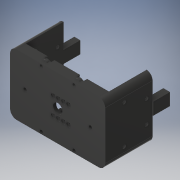
# Autodesk Inventor part: GA03
Saved by Autodesk Inventor 2017 (Build 210142000, 142)
## iProperties
Created: 2018-10-24
Part Number: GA03
Material: ABS Plastic
Document SubType Name: Modeling
Designer: Dell
Density: 1.06 g/cm^3
Appearance: Smooth - Black
Author: Dell
Autodesk Inventor part; units mm, degrees
ref_plane "YZ Plane" through (0, 0, 0) normal (1, 0, 0) x (0, 1, 0)
ref_plane "XZ Plane" through (0, 0, 0) normal (0, 1, 0) x (-1, 0, 0)
ref_plane "XY Plane" through (0, 0, 0) normal (0, 0, 1) x (1, 0, 0)
sketch "Sketch1" plane through (0, 0, 0) normal (0, 0, 1) x (1, 0, 0)
  line L0 (0, 0) -> (150, 0)
  line L1 (150, 0) -> (150, 96.9948)
  line L2 (150, 96.9948) -> (0, 96.9948)
  line L3 (0, 96.9948) -> (0, 0)
  dimension "d0" = 150
  dimension "d1" = 96.9948
  constraints: 8 end point, 2 parallel, 1 horizontal, 1 perpendicular
  measures "d0" distance of L2.end L1.end
  measures "d1" distance of L1.end L0.end
extrude "Extrusion1" add sketch "Sketch1" along normal blind 15
sketch "Sketch2" plane through (0, 0, 0) normal (0, 0, -1) x (-1, 0, 0)
  line L0 (0, 96.9948) -> (0, 0) projected
  line L1 (0, 0) -> (-150, 0) projected
  line L2 (0, 96.9948) -> (-10, 96.9948)
  line L3 (-10, 96.9948) -> (-10, 0)
  line L4 (-10, 0) -> (0, 0)
  line L5 (0, 0) -> (0, 96.9948)
  line L6 (-150, 96.9948) -> (0, 96.9948) projected
  line L7 (-150, 96.9948) -> (-140, 96.9948)
  line L8 (-140, 96.9948) -> (-140, 0)
  line L9 (-140, 0) -> (-150, 0)
  line L10 (-150, 0) -> (-150, 96.9948)
  dimension "d4" = 10
  dimension "d5" = 10
  constraints: 16 end point, 4 parallel, 2 horizontal, 2 perpendicular, 2 point on line
  measures "d4" distance between parallel lines of L3 L0
  measures "d5" distance between parallel lines of L10 L8
extrude "Extrusion2" add sketch "Sketch2" along normal blind 60 contours L0 L1 L3 L2 | L8 L1 L10 L6
sketch "Sketch3" plane through (150, 0, 15) normal (1, 0, 0) x (0, 0, -1)
  circle A0 centre (65, 65.9974) radius 2.5
  circle A1 centre (65, 30.9974) radius 2.5
  line L0 (75, 0) -> (75, 96.9948) projected
  line L1 (65, 65.9974) -> (65, 30.9974) construction
  point P0 (15, 0)
  point P1 (65, 48.4974)
  point P2 (75, 48.4974)
  dimension "d8" = 5
  dimension "d9" = 5
  dimension "d10" = 10
  dimension "d11" = 35
  constraints: 2 centre point, 2 end point, 2 midpoint, 1 horizontal alignment, 1 vertical
  measures "d8" diameter of A0
  measures "d9" diameter of A1
  measures "d10" distance from line of L0 L1.start
  measures "d11" distance of L1.end L1.start
extrude "Extrusion3" cut sketch "Sketch3" against normal through all
sketch "Sketch4" plane through (0, 0, 15) normal (0, 0, 1) x (1, 0, 0)
  line L0 (0, 0) -> (150, 0) projected
  line L1 (150, 0) -> (150, 96.9948) projected
  line L2 (150, 96.9948) -> (0, 96.9948) projected
  line L3 (0, 96.9948) -> (0, 0) projected
  line L4 (149, 1) -> (1, 1)
  line L5 (1, 1) -> (1, 95.9948)
  line L6 (1, 95.9948) -> (149, 95.9948)
  line L7 (149, 95.9948) -> (149, 1)
  dimension "d14" = 1
  constraints: 8 end point, 3 other
  measures "d14" distance between parallel lines of L0 L4
extrude "Extrusion4" cut sketch "Sketch4" against normal through all
sketch "Sketch5" plane through (1, 1, 15) normal (-1, 0, 0) x (0, 0, 1)
  line L0 (-75, 0) -> (-75, 94.9948) projected
  line L1 (-75, 94.9948) -> (-15, 94.9948) projected
  line L2 (-75, 0) -> (-74, 0)
  line L3 (-74, 0) -> (-74, 94.9948)
  line L4 (-74, 94.9948) -> (-75, 94.9948)
  line L5 (-75, 94.9948) -> (-75, 0)
  point P0 (-15, -1)
  dimension "d17" = 1
  constraints: 8 end point, 2 parallel, 1 horizontal, 1 perpendicular, 1 point on line
  measures "d17" distance between parallel lines of L0 L3
extrude "Extrusion5" cut sketch "Sketch5" against normal through all
sketch "Sketch6" plane through (0, 0, 0) normal (0, 0, -1) x (-1, 0, 0)
  line L0 (-10, 95.9948) -> (-140, 95.9948) projected
  line L1 (-140, 95.9948) -> (-140, 1) projected
  line L2 (-140, 1) -> (-10, 1) projected
  line L3 (-10, 1) -> (-10, 95.9948) projected
  line L4 (-15, 6) -> (-135, 6)
  line L5 (-135, 6) -> (-135, 90.9948)
  line L6 (-135, 90.9948) -> (-15, 90.9948)
  line L7 (-15, 90.9948) -> (-15, 6)
  line L8 (-10, 1) -> (-10, 95.9948) projected
  circle A0 centre (-75, 48.4974) radius 2.5
  circle A1 centre (-126, 48.4974) radius 2.5
  circle A2 centre (-100.5, 4.3301) radius 2.5
  circle A3 centre (-49.5, 4.3301) radius 2.5
  circle A4 centre (-24, 48.4974) radius 2.5
  circle A5 centre (-49.5, 92.6647) radius 2.5
  circle A6 centre (-100.5, 92.6647) radius 2.5
  circle A7 centre (-126, 48.4974) radius 5
  circle A8 centre (-100.5, 4.3301) radius 5
  circle A9 centre (-49.5, 4.3301) radius 5
  circle A10 centre (-24, 48.4974) radius 5
  circle A11 centre (-49.5, 92.6647) radius 5
  circle A12 centre (-100.5, 92.6647) radius 5
  point P0 (0, 0)
  point P1 (-75, 6)
  point P2 (-75, 1)
  point P3 (-15, 48.4974)
  point P4 (-10, 48.4974)
  dimension "d20" = 5
  dimension "d21" = 5
  dimension "d22" = 5
  dimension "d23" = 5
  dimension "d26" = 51
  dimension "d29" = 360
  dimension "d31" = 10
  dimension "d34" = 360
  constraints: 13 centre point, 8 end point, 4 midpoint, 3 horizontal alignment, 2 coincident, 2 parallel, 2 vertical alignment, 1 horizontal, 1 perpendicular, 26 other
  measures "d20" distance between parallel lines of L2 L4
  measures "d21" distance between parallel lines of L3 L7
  measures "d22" diameter of A0
  measures "d23" diameter of A1
  measures "d26" distance of A1.centre A0.centre
  measures "d31" diameter of A7
extrude "Extrusion6" cut sketch "Sketch6" against normal blind 10 contours A11 L6 L7 L4 A9 A8 L5 A12 | L6 A5 A11 | A12 L6 A6 | L6 A5 | A9 L4 A3 | A6 L6 | A3 L4 | L4 A2 A8 | L4 A2 | A0 picked at (-49.9702, 90.8634) picked at (-100.0298, 90.8634) picked at (-49.0298, 6.1314) picked at (-100.7933, 6.2234)
extrude "Extrusion7" cut sketch "Sketch6" against normal through all contours A5 L6 | L6 A5 | A6 L6 | L6 A6 | A3 L4 | L4 A3 | A2 L4 | L4 A2 | A1 | A4
extrude "Extrusion8" add sketch "Sketch6" against normal blind 10 contours A11 L6 A5 L0 | L0 A11 | A9 L2 | L2 A9 L4 A3 | A12 L6 A6 L0 | L0 A12 | L6 A5 A11 | A12 L6 A6 | A8 L2 | L2 A8 L4 A2 | A9 L4 A3 | L4 A2 A8
sketch "Sketch7" plane through (0, 0, 10) normal (0, 0, -1) x (-1, 0, 0)
  line L0 (-92, 61.9974) -> (-68, 61.9974) construction
  line L1 (-68, 61.9974) -> (-68, 34.9974) construction
  line L2 (-68, 34.9974) -> (-92, 34.9974) construction
  line L3 (-92, 34.9974) -> (-92, 61.9974) construction
  circle A0 centre (-92, 61.9974) radius 1.5
  circle A1 centre (-92, 34.9974) radius 1.5
  circle A2 centre (-68, 34.9974) radius 1.5
  circle A3 centre (-68, 61.9974) radius 1.5
  circle A4 centre (-84, 61.9974) radius 1.5
  circle A5 centre (-76, 61.9974) radius 1.5
  circle A6 centre (-84, 34.9974) radius 1.5
  circle A7 centre (-76, 34.9974) radius 1.5
  circle A8 centre (-24, 48.4974) radius 2.5 projected
  line L4 (-149, 1) -> (-149, 95.9948) projected
  point P0 (0, 0)
  point P1 (-92, 48.4974)
  point P2 (-80, 61.9974)
  dimension "d42" = 24
  dimension "d43" = 27
  dimension "d44" = 3
  dimension "d45" = 3
  dimension "d46" = 3
  dimension "d47" = 3
  dimension "d48" = 3
  dimension "d49" = 3
  dimension "d50" = 3
  dimension "d51" = 3
  dimension "d52" = 8
  dimension "d53" = 8
  dimension "d55" = 57
  constraints: 8 centre point, 8 end point, 4 coincident, 4 point on line, 2 midpoint, 2 parallel, 2 vertical alignment, 1 horizontal, 1 horizontal alignment, 1 perpendicular
  measures "d42" distance of L2.start L2.end
  measures "d43" distance of L0.end L2.start
  measures "d44" diameter of A0
  measures "d45" diameter of A1
  measures "d46" diameter of A2
  measures "d47" diameter of A3
  measures "d48" diameter of A4
  measures "d49" diameter of A5
  measures "d50" diameter of A6
  measures "d51" diameter of A7
  measures "d52" distance of L2.start A7.centre
  measures "d53" distance of L2.end A6.centre
  measures "d55" distance between parallel lines of L4 L3
extrude "Extrusion9" cut sketch "Sketch7" against normal through all contours A0 | A1 | A2 | A3 | A4 | A5 | A6 | A7
sketch "Sketch8" plane through (0, 0, 10) normal (0, 0, -1) x (-1, 0, 0)
  circle A0 centre (-68, 34.9974) radius 1.5 projected
  circle A1 centre (-76, 34.9974) radius 1.5 projected
  circle A2 centre (-84, 34.9974) radius 1.5 projected
  circle A3 centre (-92, 34.9974) radius 1.5 projected
  circle A4 centre (-92, 61.9974) radius 1.5 projected
  circle A5 centre (-84, 61.9974) radius 1.5 projected
  circle A6 centre (-76, 61.9974) radius 1.5 projected
  circle A7 centre (-68, 61.9974) radius 1.5 projected
  circle A8 centre (-68, 34.9974) radius 3.5
  circle A9 centre (-76, 34.9974) radius 3.5
  circle A10 centre (-84, 34.9974) radius 3.5
  circle A11 centre (-92, 34.9974) radius 3.5
  circle A12 centre (-92, 61.9974) radius 3.5
  circle A13 centre (-84, 61.9974) radius 3.5
  circle A14 centre (-76, 61.9974) radius 3.5
  circle A15 centre (-68, 61.9974) radius 3.5
  point P0 (0, 0)
  dimension "d58" = 7
  dimension "d59" = 7
  dimension "d60" = 7
  dimension "d61" = 7
  dimension "d62" = 7
  dimension "d63" = 7
  dimension "d64" = 7
  dimension "d65" = 7
  constraints: 8 centre point, 8 coincident
  measures "d58" diameter of A8
  measures "d59" diameter of A9
  measures "d60" diameter of A10
  measures "d61" diameter of A11
  measures "d62" diameter of A12
  measures "d63" diameter of A13
  measures "d64" diameter of A14
  measures "d65" diameter of A15
extrude "Extrusion10" add sketch "Sketch8" along normal blind 8
sketch "Sketch10" plane through (0, 0, 0) normal (0, 0, -1) x (-1, 0, 0)
  circle A0 centre (-126, 48.4974) radius 2.5 projected
  circle A1 centre (-24, 48.4974) radius 2.5 projected
  circle A2 centre (-49.5, 4.3301) radius 2.5 projected
  circle A3 centre (-100.5, 92.6647) radius 2.5 projected
  circle A4 centre (-49.5, 92.6647) radius 2.5 projected
  circle A5 centre (-100.5, 4.3301) radius 2.5 projected
  circle A6 centre (-49.5, 4.3301) radius 6.5
  circle A7 centre (-100.5, 4.3301) radius 6.5
  circle A8 centre (-126, 48.4974) radius 6.5
  circle A9 centre (-100.5, 92.6647) radius 6.5
  circle A10 centre (-49.5, 92.6647) radius 5 projected
  circle A11 centre (-49.5, 92.6647) radius 6.5
  circle A12 centre (-24, 48.4974) radius 6.5
  point P0 (0, 0)
  point P1 (-44.7871, 90.9948)
  point P2 (-54.2129, 90.9948)
  dimension "d69" = 13
  dimension "d70" = 13
  dimension "d71" = 13
  dimension "d72" = 13
  dimension "d73" = 13
  dimension "d74" = 13
  constraints: 6 centre point, 6 coincident
  measures "d69" diameter of A6
  measures "d70" diameter of A7
  measures "d71" diameter of A8
  measures "d72" diameter of A9
  measures "d73" diameter of A11
  measures "d74" diameter of A12
extrude "Extrusion11" cut sketch "Sketch10" against normal blind 5 contours A0 | A1 | A2 | A3 | A4 | A5 | A6 | A7 | A8 | A9 | A10 | A11 | A12
sketch "Sketch12" plane through (0, 0, 15) normal (0, 0, 1) x (1, 0, 0)
  circle A0 centre (84, 61.9974) radius 1.5 projected
  circle A1 centre (68, 61.9974) radius 1.5 projected
  circle A2 centre (76, 61.9974) radius 1.5 projected
  circle A3 centre (92, 61.9974) radius 1.5 projected
  circle A4 centre (92, 34.9974) radius 1.5 projected
  circle A5 centre (84, 34.9974) radius 1.5 projected
  circle A6 centre (76, 34.9974) radius 1.5 projected
  circle A7 centre (68, 34.9974) radius 1.5 projected
  circle A8 centre (68, 61.9974) radius 3.5
  circle A9 centre (76, 61.9974) radius 1.5 projected
  circle A10 centre (76, 61.9974) radius 3.5
  circle A11 centre (84, 61.9974) radius 3.5
  circle A12 centre (92, 61.9974) radius 1.5 projected
  circle A13 centre (92, 61.9974) radius 3.5
  circle A14 centre (92, 34.9974) radius 3.5
  circle A15 centre (84, 34.9974) radius 3.5
  circle A16 centre (76, 34.9974) radius 3.5
  circle A17 centre (68, 34.9974) radius 3.5
  point P0 (0, 0)
  dimension "d77" = 7
  dimension "d78" = 7
  dimension "d79" = 7
  dimension "d80" = 7
  dimension "d81" = 7
  dimension "d82" = 7
  dimension "d83" = 7
  dimension "d84" = 7
  constraints: 8 centre point, 8 coincident
  measures "d77" diameter of A8
  measures "d78" diameter of A10
  measures "d79" diameter of A11
  measures "d80" diameter of A13
  measures "d81" diameter of A14
  measures "d82" diameter of A15
  measures "d83" diameter of A16
  measures "d84" diameter of A17
extrude "Extrusion12" cut sketch "Sketch12" against normal blind 2 contours A0 | A1 | A2 | A3 | A4 | A5 | A6 | A7 | A8 | A10 | A11 | A13 | A14 | A15 | A16 | A17
sketch "Sketch13" plane through (1, 1, 15) normal (-1, 0, 0) x (0, 0, 1)
  line L0 (-74, 94.9948) -> (-74, 0) projected
  line L1 (-74, 37.9974) -> (-100, 37.9974)
  line L2 (-100, 37.9974) -> (-100, 56.9974)
  line L3 (-100, 56.9974) -> (-74, 56.9974)
  line L4 (-74, 56.9974) -> (-74, 37.9974)
  point P0 (-15, -1)
  point P1 (-74, 47.4974)
  dimension "d87" = 19
  dimension "d88" = 26
  constraints: 8 end point, 2 midpoint, 2 parallel, 1 horizontal, 1 perpendicular, 1 point on line
  measures "d87" distance of L1.end L2.end
  measures "d88" distance of L1.start L1.end
extrude "Extrusion13" add sketch "Sketch13" against normal blind 9
sketch "Sketch14" plane through (0, 0, 10) normal (0, 0, -1) x (-1, 0, 0)
  line L0 (-10, 95.9948) -> (-140, 95.9948) projected
  line L1 (-149, 1) -> (-149, 95.9948) projected
  circle A0 centre (-75, 48.4974) radius 7.5
  point P0 (0, 0)
  point P1 (-55.0821, 95.9948)
  point P2 (-94.9179, 95.9948)
  point P3 (-149, 48.4974)
  point P4 (-75, 95.9948)
  dimension "d92" = 15
  constraints: 2 midpoint, 1 centre point, 1 horizontal alignment, 1 vertical alignment
  measures "d92" diameter of A0
extrude "Extrusion14" cut sketch "Sketch14" against normal through all
fillet "Fillet1" radius 10 4 edges at (1, 95.9948, -22) (149, 95.9948, -22) (149, 1, -22) (1, 1, -22)
sketch "Sketch15" plane through (140, 1.0501, 0) normal (-1, 0, 0) x (0, 0, 1)
  line L0 (15, 9.9499) -> (-59, 9.9499) projected
  line L1 (15, 84.9447) -> (15, 9.9499) projected
  line L2 (-59, 84.9447) -> (15, 84.9447) projected
  line L3 (-59, 84.9447) -> (-59, 56.9473) projected
  line L4 (-59, 56.9473) -> (-85, 56.9473) projected
  line L5 (-85, 56.9473) -> (-85, 37.9473) projected
  line L6 (-85, 37.9473) -> (-59, 37.9473) projected
  line L7 (-59, 37.9473) -> (-59, 9.9499) projected
  circle A0 centre (-50, 29.9473) radius 2.5 projected
  circle A1 centre (-50, 64.9473) radius 2.5 projected
  line L8 (-59, 37.9473) -> (-59, 56.9473)
  line L9 (-59, 94.8946) -> (-59, 0) projected
  point P0 (0, -1.0501)
  constraints: 2 end point, 1 collinear
extrude "Extrusion15" add sketch "Sketch15" against normal blind 10 contours L6 L5 L4 L8
sketch "Sketch16" plane through (149, 11, 15) normal (1, 0, 0) x (0, 0, -1)
  line L0 (15, 84.9447) -> (15, -9.9499) construction
  circle A0 centre (30, 67.4974) radius 2.5
  circle A1 centre (30, 7.4974) radius 2.5
  line L1 (30, 67.4974) -> (30, 7.4974) construction
  point P0 (15, -11)
  point P1 (30, 37.4974)
  point P2 (15, 37.4974)
  dimension "d98" = 5
  dimension "d99" = 5
  dimension "d100" = 60
  dimension "d101" = 15
  constraints: 2 centre point, 2 end point, 2 midpoint, 1 horizontal alignment, 1 vertical
  measures "d98" diameter of A0
  measures "d99" diameter of A1
  measures "d100" distance of L1.start L1.end
  measures "d101" distance between parallel lines of L0 L1
extrude "Extrusion16" cut sketch "Sketch16" against normal through all
body "Solid1"
